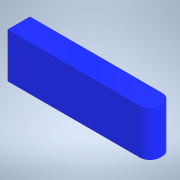
# Autodesk Inventor part: akum12v
Saved by Autodesk Inventor 2022 (Build 260153000, 153)
## iProperties
Created: 2023-05-26
Part Number: akum12v
Material: Типовые
Document SubType Name: Modeling
Designer: korsh624
Density: 1 g/cm^3
Appearance: Синий — малярная краска — глянцевая
Author: korsh624
Autodesk Inventor part; units mm, degrees
ref_plane "YZ Plane" through (0, 0, 0) normal (1, 0, 0) x (0, 1, 0)
ref_plane "XZ Plane" through (0, 0, 0) normal (0, 1, 0) x (-1, 0, 0)
ref_plane "XY Plane" through (0, 0, 0) normal (0, 0, 1) x (1, 0, 0)
sketch "Эскиз1" plane through (0, 0, 0) normal (0, 0, 1) x (1, 0, 0)
  line L0 (74.0863, 5.032) -> (74.0863, 52.032) projected
  line L1 (81.155, -20.903) -> (-58.845, -20.903)
  line L2 (-58.845, -20.903) -> (-58.845, -64.903)
  line L3 (-58.845, -64.903) -> (81.155, -64.903)
  line L4 (81.155, -64.903) -> (81.155, -20.903)
  point P0 (0, 0)
  dimension "d0" = 44
  dimension "d1" = 140
  constraints: 8 end point, 2 parallel, 1 horizontal, 1 perpendicular
  measures "d0" distance of L3.end L1.start
  measures "d1" distance of L1.start L1.end
extrude "Выдавливание1" add sketch "Эскиз1" along normal blind 22
fillet "Сопряжение1" radius 10 2 edges at (81.155, -42.903, 22) (81.155, -42.903, 0)
